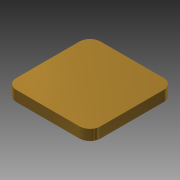
# Autodesk Inventor part: termination_closing
Saved by Autodesk Inventor 2014 SP1 (Build 180222100, 222)
## iProperties
Created: 2016-10-15
Part Number: termination_closing
Material: Brass, Soft Yellow
Document SubType Name: Modeling
Designer: tguillod
Density: 8.47 g/cm^3
Appearance: Brass - Satin
Author: tguillod
Autodesk Inventor part; units mm, degrees
ref_plane "YZ Plane" through (0, 0, 0) normal (1, 0, 0) x (0, 1, 0)
ref_plane "XZ Plane" through (0, 0, 0) normal (0, 1, 0) x (-1, 0, 0)
ref_plane "XY Plane" through (0, 0, 0) normal (0, 0, 1) x (1, 0, 0)
sketch "Sketch1" plane through (0, 0, 0) normal (0, 0, 1) x (1, 0, 0)
  line L0 (1, 0) -> (7, 0)
  line L1 (8, 1) -> (8, 7)
  line L2 (7, 8) -> (1, 8)
  line L3 (0, 7) -> (0, 1)
  arc A0 (1, 8) -> (0, 7) centre (1, 7) ccw
  arc A1 (7, 0) -> (8, 1) centre (7, 1) ccw
  arc A2 (8, 7) -> (7, 8) centre (7, 7) ccw
  arc A3 (0, 1) -> (1, 0) centre (1, 1) ccw
  point P0 (0, 0)
  point P1 (8, 8)
  point P2 (8, 0)
  point P3 (0, 8)
  dimension "d0" = 8
  dimension "d1" = 8
  dimension "d2" = 1
  constraints: 8 end point, 8 point on circle, 8 point on line, 8 tangent, 4 centre point, 3 equal radius, 2 parallel, 1 horizontal, 1 perpendicular
  measures "d0" distance of point (8, 8) point (0, 8)
  measures "d1" distance of point (8, 0) point (8, 8)
  measures "d2" radius of A0
extrude "Extrusion1" add sketch "Sketch1" along normal blind 1
body "Solid1"
